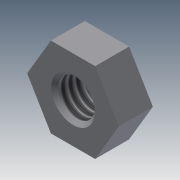
# Autodesk Inventor part: matka_m3
Saved by Autodesk Inventor 2013 (Build 170138000, 138)
## iProperties
Created: 2013-03-08
Part Number: matka_m3
Material: Generic
Document SubType Name: Modeling
Designer: idle-rug
Density: 1 g/cm^3
Author: idle-rug
Autodesk Inventor part; units mm, degrees
ref_plane "YZ Plane" through (0, 0, 0) normal (1, 0, 0) x (0, 1, 0)
ref_plane "XZ Plane" through (0, 0, 0) normal (0, 1, 0) x (-1, 0, 0)
ref_plane "XY Plane" through (0, 0, 0) normal (0, 0, 1) x (1, 0, 0)
sketch "Sketch1" plane through (0, 0, 0) normal (0, 1, 0) x (-1, 0, 0)
  line L0 (-1.5, -2.725) -> (1.5, -2.725)
  line L1 (1.5, 2.725) -> (-1.5, 2.725)
  line L2 (-1.5, -2.725) -> (-3.1106, 0)
  line L3 (-3.1106, 0) -> (-1.5, 2.725)
  line L4 (-1.5, 2.725) -> (-3.1106, 0)
  line L5 (-3.1106, 0) -> (-1.5, -2.725)
  line L6 (-1.5, -2.725) -> (1.5, -2.725)
  line L7 (-1.5, 2.725) -> (1.5, 2.725)
  line L8 (1.5, 2.725) -> (3.1106, 0)
  line L9 (1.5, -2.725) -> (3.1106, 0)
  point P0 (0, 0)
  dimension "d5" = 3
  dimension "d6" = 5.45
  constraints: 20 end point, 7 equal length, 1 horizontal
  measures "d5" distance of L1.end L1.start
  measures "d6" distance of L1.start L0.end
extrude "Extrusion1" add sketch "Sketch1" along normal blind 2.3
sketch "Sketch2" plane through (0, 2.3, 0) normal (0, 1, 0) x (1, 0, 0)
  point P0 (0, 0)
hole "Hole1" at (0, 2.3, 0) direction (0, -1, 0) diameter 2.459 depth 8 thread size "M3x0.5" class "6H" standard "ANSI Metric M Profile"
chamfer "Chamfer1" distance 0.25 angle 45 1 edges at (0, 2.3, -1.2295)
chamfer "Chamfer2" distance 0.25 angle 45 1 edges at (0, 0, -1.2295)
body "Solid1"
